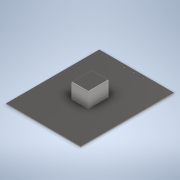
# Autodesk Inventor part: top_sensor
Saved by Autodesk Inventor 2020 (Build 240168000, 168)
## iProperties
Created: 2020-05-04
Part Number: top_sensor
Material: Generic
Document SubType Name: Modeling
Designer: Abbas
Density: 1 g/cm^3
Appearance: Default
Author: Abbas
Autodesk Inventor part; units mm, degrees
ref_plane "YZ Plane" through (0, 0, 0) normal (1, 0, 0) x (0, 1, 0)
ref_plane "XZ Plane" through (0, 0, 0) normal (0, 1, 0) x (-1, 0, 0)
ref_plane "XY Plane" through (0, 0, 0) normal (0, 0, 1) x (1, 0, 0)
sketch "Sketch1" plane through (0, 0, 0) normal (0, 1, 0) x (-1, 0, 0)
  line L0 (100, 125) -> (-100, 125)
  line L1 (-100, 125) -> (-100, -125)
  line L2 (-100, -125) -> (100, -125)
  line L3 (100, -125) -> (100, 125)
  line L4 (100, 125) -> (-100, -125) construction
  line L5 (-100, 125) -> (100, -125) construction
  circle A0 centre (0, 12.655) radius 8.2
  circle A1 centre (0, -12.655) radius 8.2
  line L6 (10.65, 6) -> (6.0435, 6)
  line L7 (6.0435, 6) -> (6.0435, -6)
  line L8 (6.0435, -6) -> (10.65, -6)
  line L9 (10.65, -6) -> (10.65, 6)
  line L10 (10.65, 6) -> (6.0435, -6) construction
  line L11 (6.0435, 6) -> (10.65, -6) construction
  circle A2 centre (0, -117) radius 1.875
  circle A3 centre (-25.8, -117) radius 1.875
  circle A4 centre (25.8, -117) radius 1.875
  point P0 (0, 0)
  dimension "d0" = 200
  dimension "d1" = 250
  dimension "d2" = 16.4
  dimension "d3" = 16.4
  dimension "d7" = 4.6065
  dimension "d8" = 12
  dimension "d14" = 3.75
  dimension "d15" = 3.75
  dimension "d16" = 3.75
  dimension "d17" = 8
  dimension "d18" = 8
  dimension "d19" = 8
  dimension "d20" = 25.8
  dimension "d21" = 25.8
  constraints: 24 end point, 5 centre point, 4 parallel, 2 horizontal, 2 midpoint, 2 perpendicular
  measures "d0" distance of L2.end L1.end
  measures "d1" distance of L1.end L0.end
  measures "d2" diameter of A0
  measures "d3" diameter of A1
  measures "d7" distance of L8.end L7.end
  measures "d8" distance of L7.end L6.end
  measures "d14" diameter of A2
  measures "d15" diameter of A3
  measures "d16" diameter of A4
  measures "d17" distance from line of L2 A2.centre
  measures "d18" distance from line of L2 A4.centre
  measures "d19" distance from line of L2 A3.centre
  measures "d20" distance of A4.centre A2.centre
  measures "d21" distance of A3.centre A2.centre
extrude "Extrusion1" add sketch "Sketch1" along normal blind 3
sketch "Sketch2" plane through (0, 3, 0) normal (0, 1, 0) x (1, 0, 0)
  line L0 (-20, 25) -> (20, 25)
  line L1 (20, 25) -> (20, -25)
  line L2 (20, -25) -> (-20, -25)
  line L3 (-20, -25) -> (-20, 25)
  line L4 (-20, 25) -> (20, -25) construction
  line L5 (20, 25) -> (-20, -25) construction
  line L6 (-23, 28) -> (23, 28)
  line L7 (23, 28) -> (23, -28)
  line L8 (23, -28) -> (-23, -28)
  line L9 (-23, -28) -> (-23, 28)
  line L10 (-23, 28) -> (23, -28) construction
  line L11 (23, 28) -> (-23, -28) construction
  point P0 (0, 0)
  dimension "d24" = 40
  dimension "d25" = 50
  dimension "d26" = 46
  dimension "d27" = 56
  constraints: 24 end point, 4 midpoint, 4 parallel, 2 horizontal, 2 perpendicular
  measures "d24" distance of L1.end L2.end
  measures "d25" distance of L0.end L1.end
  measures "d26" distance of L7.end L8.end
  measures "d27" distance of L6.end L7.end
extrude "Extrusion2" add sketch "Sketch2" along normal blind 37
sketch "Sketch3" plane through (0, 40, 0) normal (0, 1, 0) x (1, 0, 0)
  line L0 (-23, -28) -> (23, -28) projected
  line L1 (-23, 28) -> (23, 28)
  line L2 (23, 28) -> (23, -28)
  line L3 (23, -28) -> (-23, -28)
  line L4 (-23, -28) -> (-23, 28)
  line L5 (-23, 28) -> (23, -28) construction
  line L6 (23, 28) -> (-23, -28) construction
  point P0 (0, 0)
  constraints: 12 end point, 2 midpoint, 2 parallel, 1 horizontal, 1 perpendicular
extrude "Extrusion3" add sketch "Sketch3" along normal blind 3
fillet "Fillet1" radius 2 8 edges at (0, 43, 28) (23, 43, 0) (0, 43, -28) (-23, 43, 0) (-23, 23, 28) (23, 23, 28) (23, 23, -28) (-23, 23, -28)
body "Solid1"
